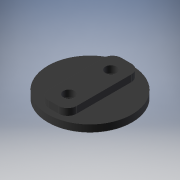
# Autodesk Inventor part: baseplate
Saved by Autodesk Inventor 2019.3 (Build 233278000, 278)
## iProperties
Created: 2019-04-10
Part Number: baseplate
Material: Generic
Document SubType Name: Modeling
Designer: peter
Density: 1 g/cm^3
Appearance: Default
Author: peter
Autodesk Inventor part; units mm, degrees
ref_plane "YZ Plane" through (0, 0, 0) normal (1, 0, 0) x (0, 1, 0)
ref_plane "XZ Plane" through (0, 0, 0) normal (0, 1, 0) x (-1, 0, 0)
ref_plane "XY Plane" through (0, 0, 0) normal (0, 0, 1) x (1, 0, 0)
sketch "Sketch1" plane through (0, 0, 0) normal (0, 1, 0) x (-1, 0, 0)
  circle A0 centre (0, 0) radius 15
  line L0 (0, 0) -> (0, -7.5) construction
  line L1 (0, -7.5) -> (0, 7.5) construction
  circle A1 centre (0, 7.5) radius 3.2
  circle A2 centre (0, -7.5) radius 3.2
  dimension "d0" = 30
  dimension "d1" = 7.5
  dimension "d2" = 15
  dimension "d3" = 6.4
  dimension "d4" = 6.4
  constraints: 4 end point, 3 centre point, 3 coincident, 2 vertical
  measures "d0" diameter of A0
  measures "d1" distance of L0.start L0.end
  measures "d2" distance of L0.end L1.end
  measures "d3" diameter of A1
  measures "d4" diameter of A2
extrude "Extrusion1" add sketch "Sketch1" along normal blind 2.5
sketch "Sketch2" plane through (0, 2.5, 0) normal (0, 1, 0) x (1, 0, 0)
  line L0 (0, 0) -> (-5, 0) construction
  line L1 (-5, 0) -> (-5, -10) construction
  line L2 (-2, -13) -> (0, -13) construction
  line L3 (0, -13) -> (0, 0) construction
  line L4 (-1.8, -13) -> (1.8, -13)
  line L5 (5, -9.8) -> (5, 9.8)
  line L6 (1.8, 13) -> (-1.8, 13)
  line L7 (-5, 9.8) -> (-5, -9.8)
  circle A0 centre (0, -7.5) radius 3.2 projected
  circle A1 centre (0, 7.5) radius 3.2 projected
  arc A2 (-5, -9.8) -> (-1.8, -13) centre (-1.8, -9.8) ccw
  arc A3 (1.8, -13) -> (5, -9.8) centre (1.8, -9.8) ccw
  arc A4 (5, 9.8) -> (1.8, 13) centre (1.8, 9.8) ccw
  arc A5 (-1.8, 13) -> (-5, 9.8) centre (-1.8, 9.8) ccw
  circle A6 centre (0, -7.5) radius 2.05
  circle A7 centre (0, 7.5) radius 2.05
  point P0 (-5, -13)
  point P1 (5, 13)
  point P2 (5, -13)
  point P3 (-5, 13)
  dimension "d7" = 5
  dimension "d8" = 13
  dimension "d9" = 10
  dimension "d10" = 26
  dimension "d12" = 3.2
  dimension "d13" = 4.1
  dimension "d14" = 4.1
  constraints: 16 end point, 10 point on line, 8 point on circle, 8 tangent, 6 centre point, 4 parallel, 3 equal radius, 2 coincident, 2 horizontal, 2 perpendicular
  measures "d7" distance of L2.end point (-5, -13)
  measures "d8" distance of point (-5, -13) L0.end
  measures "d9" distance of point (-5, 13) point (5, 13)
  measures "d10" distance of point (5, 13) point (5, -13)
  measures "d12" radius of A2
  measures "d13" diameter of A6
  measures "d14" diameter of A7
extrude "Extrusion2" add sketch "Sketch2" along normal blind 2.5 contours A2 L7 A5 L6 A4 L5 A3 L4 | A0 | A1
body "Solid1"
